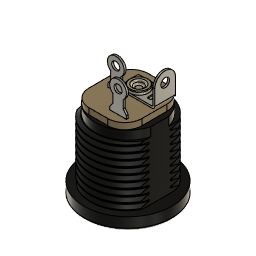
DC jack (Autodesk Fusion 360 design; units mm, degrees)
Autodesk Fusion 360 part; units mm, degrees
note: some values were not read from the file. Chosen so that the rebuilt part matches the saved one: which pieces of a blend or face edit are solid. Set by a fixed rule: which sketch regions a step uses.
sketch "Sketch1" plane through (0, 0, 0) normal (0, 0, 1) x (1, 0, 0)
  circle A0 centre (0, 0) radius 7.05
  line L0 (0, 0) -> (0, 7.05) construction
  circle A1 centre (0, 1.75) radius 3.2
  dimension "d1" = 14.1
  dimension "d2" = 6.4
  dimension "d3" = 2.1
  constraint coincident A0.centre L0.start
  constraint coincident A0 L0.end
  constraint vertical L0
  constraint coincident L0 A1.centre
  measures "d1" diameter of A0
  measures "d2" diameter of A1
  measures "d3" distance of L0.end A1
extrude "Extrude1" add sketch "Sketch1" along normal blind 2 contours A0 | A1 makes body 1
sketch "Sketch2" plane through (0, 0, 2) normal (0, 0, 1) x (-1, 0, 0)
  circle A0 centre (0, 0) radius 6
  constraint coincident A0.centre origin
extrude "Extrude2" add sketch "Sketch2" along normal blind 9.4 bodies 1
sketch "Sketch3" plane through (0, 0, 11.4) normal (0, 0, 1) x (-1, 0, 0)
  circle A0 centre (0, 0) radius 5.3
  dimension "d8" = 10.6
  constraint coincident A0.centre origin
  measures "d8" diameter of A0
extrude "Extrude3" add sketch "Sketch3" along normal blind 1.4 bodies 1
extrude "Extrude4" cut sketch "Sketch1" along normal blind 10.8 contours A1 bodies 1
thread "Thread1" "ISO Metric profile 12.0 M12x1 6g" major diameter 11.884 minor diameter 10.7405 pitch 1 angle 60 modelled right hand crest width 0.1426 on face at (-5.9925, 0.2991, 8.2667) crest through (-5.942, 0, 1.75) on bodies 1
sketch "Sketch4" plane through (0, 0, 12.8) normal (0, 0, 1) x (-1, 0, 0)
  line L0 (0, 0) -> (-5.1, 0) construction
  line L1 (0, 0) -> (0, -3.5) construction
  line L2 (-5.1, 0) -> (-5.1, -6.5)
  line L3 (-5.1, -6.5) -> (-9, -6.5)
  line L4 (-9, -6.5) -> (-9, 7.5)
  line L5 (-9, 7.5) -> (-5.1, 7.5)
  line L6 (-5.1, 7.5) -> (-5.1, 0)
  line L7 (5.1, 0) -> (5.1, -6.5)
  line L8 (5.1, -6.5) -> (9, -6.5)
  line L9 (9, -6.5) -> (9, 7.5)
  line L10 (9, 7.5) -> (5.1, 7.5)
  line L11 (5.1, 7.5) -> (5.1, 0)
  dimension "d13" = 5.1
  constraint coincident L0.start L1.start
  constraint horizontal L0
  constraint perpendicular L0 L1
  constraint perpendicular L0 L2
  constraint perpendicular L2 L3
  constraint perpendicular L3 L4
  constraint perpendicular L2 L5
  constraint perpendicular L0 L6
  constraint symmetric L0.end L1 L7.start
  constraint symmetric L1 L2.end L7.end
  constraint symmetric L1 L3.end L8.end
  constraint symmetric L1 L4.end L9.end
  constraint symmetric L1 L5.end L10.end
  measures "d13" distance of L0.start L0.end
extrude "Extrude5" cut sketch "Sketch4" against normal up to surface (10.8 mm away) bodies 1
sketch "Sketch5" plane through (0, 0, 12.8) normal (0, 0, 1) x (-1, 0, 0)
  circle A0 centre (0, -1.75) radius 3.2
  circle A1 centre (0, -1.75) radius 1
  line L0 (3.58, 0.05) -> (-3.58, 0.05)
  line L1 (0, -1.75) -> (0, 4.5) construction
  line L2 (2.17, 4.05) -> (2.17, 3.35)
  line L3 (-2.17, 4.05) -> (-2.17, 3.35)
  line L4 (3.58, 3.35) -> (2.17, 3.35)
  line L5 (-2.17, 3.35) -> (-3.58, 3.35)
  line L6 (-0.3, 4.05) -> (-0.3, 3.35)
  line L7 (0.3, 3.35) -> (0.3, 4.05)
  line L8 (-0.3, 3.35) -> (0.3, 3.35)
  line L9 (2.17, 4.05) -> (0.3, 4.05)
  line L10 (-0.3, 4.05) -> (-2.17, 4.05)
  line L11 (3.58, 3.35) -> (3.58, 3.05)
  line L12 (-3.58, 3.35) -> (-3.58, 3.05)
  line L13 (3.58, 0.05) -> (3.58, 0.35)
  line L14 (-3.58, 0.05) -> (-3.58, 0.35)
  line L15 (2.95, 0.05) -> (2.95, 3.35)
  line L16 (3.58, 0.35) -> (2.95, 0.35)
  line L17 (3.58, 3.05) -> (2.95, 3.05)
  line L18 (-3.58, 0.35) -> (-2.95, 0.35)
  line L19 (-2.95, 0.05) -> (-2.95, 3.35)
  line L20 (-3.58, 3.05) -> (-2.95, 3.05)
  dimension "d16" = 2
  dimension "d17" = 0.8
  dimension "d18" = 3.58
  dimension "d19" = 3.58
  dimension "d22" = 2.17
  dimension "d23" = 2.17
  dimension "d24" = 0.3
  dimension "d25" = 0.3
  dimension "d26" = 0.3
  dimension "d27" = 0.3
  dimension "d28" = 0.3
  dimension "d29" = 0.3
  dimension "d30" = 2.95
  constraint concentric A0 A1
  constraint horizontal L0
  constraint coincident A0.centre A1.centre
  constraint perpendicular L0 L1
  constraint parallel L0 L9
  constraint perpendicular L2 L4
  constraint coincident L3.end L4
  constraint perpendicular L3 L4
  constraint parallel L0 L4
  constraint collinear L4 L5
  constraint coincident L6.start L9
  constraint perpendicular L5 L6
  constraint perpendicular L7 L9
  constraint perpendicular L6 L8
  constraint collinear L9 L10
  constraint perpendicular L4 L11
  constraint perpendicular L5 L12
  constraint perpendicular L0 L13
  constraint perpendicular L0 L14
  constraint parallel L11 L15
  constraint perpendicular L15 L16
  constraint perpendicular L15 L17
  constraint symmetric L1 L11.end L12.end
  constraint symmetric L1 L13.end L14.end
  constraint symmetric L1 L16.end L18.end
  constraint symmetric L1 L17.end L20.end
  constraint coincident L0 L15.start
  constraint coincident L16.end L15
  constraint coincident L4 L15.end
  constraint coincident L17.end L15
  constraint coincident L0 L19.start
  constraint coincident L18.end L19
  constraint coincident L20.end L19
  measures "d16" diameter of A1
  measures "d17" distance of A1 L0
  measures "d18" distance of L0.end L1
  measures "d19" distance of L0.start L1
  measures "d22" distance of L1 L3.start
  measures "d23" distance of L1 L2.start
  measures "d24" distance of L1 L6
  measures "d25" distance of L1 L7
  measures "d26" distance of L4.start L11.end
  measures "d27" distance of L5.end L12.end
  measures "d28" distance of L0.start L13.end
  measures "d29" distance of L0.end L14.end
  measures "d30" distance of L1 L15
extrude "Extrude6" cut sketch "Sketch5" against normal blind 5.3 contours L0 L13 L15 L16 | L0 L14 L18 L19 | L4 L11 L15 L17 | L5 L12 L19 L20 bodies 1
extrude "Extrude7" cut sketch "Sketch5" against normal up to surface (10.8 mm away) contours A0 L0 | A0 L0 L2 L3 L4 L5 L6 L7 L8 L9 L10 L15 L19 picked at (0.0798, 0.5137) bodies 1
extrude "Extrude8" cut sketch "Sketch5" against normal up to surface (2 mm away) contours A1 bodies 1
fillet "Fillet1" radius 0.4 1 faces at (0.7783, -5.1149, 0) on bodies 1
sketch "Sketch6" plane through (0, -0.05, 0) normal (0, -1, 0) x (1, 0, 0)
  line L0 (-2.95, 2) -> (-2.6458, 2)
  line L1 (2.6458, 2) -> (2.95, 2)
  line L2 (-3.48, 7.5) -> (-3.044, 7.5)
  line L3 (0, 5) -> (0, 13.7) construction
  line L4 (-1.786, 9.95) -> (0, 9.95)
  line L5 (-1.8768, 9.8919) -> (-2.9532, 7.5581)
  line L6 (-3.58, 12.7) -> (-3.58, 7.6)
  arc A0 (-3.58, 7.6) -> (-3.48, 7.5) centre (-3.48, 7.6) ccw
  arc A1 (-3.044, 7.5) -> (-2.9532, 7.5581) centre (-3.044, 7.6) ccw
  arc A2 (-1.786, 9.95) -> (-1.8768, 9.8919) centre (-1.786, 9.85) ccw
  line L7 (-2.88, 12.8) -> (-2.88, 14.3)
  line L8 (-0.34, 12.8) -> (-0.34, 14.3)
  arc A3 (-3.48, 12.8) -> (-3.58, 12.7) centre (-3.48, 12.7) ccw
  line L9 (3.58, 12.7) -> (3.58, 7.6)
  arc A4 (3.58, 12.7) -> (3.48, 12.8) centre (3.48, 12.7) ccw
  arc A5 (3.48, 7.5) -> (3.58, 7.6) centre (3.48, 7.6) ccw
  line L10 (3.48, 7.5) -> (3.044, 7.5)
  arc A6 (2.9532, 7.5581) -> (3.044, 7.5) centre (3.044, 7.6) ccw
  line L11 (1.8768, 9.8919) -> (2.9532, 7.5581)
  arc A7 (1.8768, 9.8919) -> (1.786, 9.95) centre (1.786, 9.85) ccw
  line L12 (1.786, 9.95) -> (0, 9.95)
  line L13 (-5, 18.7) -> (6, 18.7) construction
  line L14 (-3.48, 12.8) -> (-2.88, 12.8)
  line L15 (-0.34, 12.8) -> (3.48, 12.8)
  line L16 (-1.61, 12.8) -> (-1.61, 18.7) construction
  circle A8 centre (-1.61, 17.35) radius 0.65
  line L17 (-2.435, 14.9814) -> (-2.435, 16.2814)
  line L18 (-2.435, 14.9814) -> (-2.88, 14.3)
  line L19 (-0.785, 14.9814) -> (-0.785, 16.2814)
  line L20 (-0.785, 14.9814) -> (-0.34, 14.3)
  arc A9 (-0.785, 16.2814) -> (-2.435, 16.2814) centre (-1.61, 17.35) ccw
  circle A10 centre (0, 11.6) radius 0.75
  point P0 (-3.58, 7.5)
  point P1 (-2.98, 7.5)
  point P2 (-1.85, 9.95)
  dimension "d39" = 0.6
  dimension "d40" = 1.85
  dimension "d42" = 0.1
  dimension "d43" = 0.1
  dimension "d44" = 0.1
  dimension "d45" = 0.7
  dimension "d46" = 2.54
  dimension "d47" = 0.1
  dimension "d50" = 1.3
  dimension "d51" = 0.7
  dimension "d54" = 1.5
  dimension "d55" = 1.5
  dimension "d56" = 0.825
  dimension "d57" = 1.3
  dimension "d58" = 1.5
  dimension "d59" = 1.2
  constraint coincident L3 L4.end
  constraint perpendicular L3 L4
  constraint perpendicular L2 L6
  constraint coincident P0 L2
  constraint coincident P0 L6
  constraint tangent L2 A0
  constraint tangent L6 A0
  constraint coincident P1 L2
  constraint coincident P1 L5
  constraint tangent L2 A1
  constraint tangent L5 A1
  constraint coincident P2 L4
  constraint coincident P2 L5
  constraint tangent L4 A2
  constraint tangent L5 A2
  constraint tangent L6 A3
  constraint symmetric L3 L4.end L12.end
  constraint symmetric L3 L2.start A5.start
  constraint symmetric L3 L6.end L9.end
  constraint symmetric L3 A0 A5
  constraint symmetric L3 L2.end L10.end
  constraint symmetric L3 L5.end A6.start
  constraint symmetric L3 A1 A6
  constraint symmetric L3 L4.start A7.end
  constraint symmetric L3 L5.start L11.start
  constraint symmetric L3 A2 A7
  constraint symmetric L3 A3.start A4.end
  constraint symmetric L3 L6.start L9.start
  constraint symmetric L3 A3 A4
  constraint horizontal L13
  constraint tangent A3 L14
  constraint perpendicular L8 L15
  constraint coincident L13 L16.end
  constraint perpendicular L13 L16
  constraint coincident L16 A8.centre
  constraint concentric A8 A9
  constraint coincident L16.end A9
  constraint vertical L17
  constraint symmetric L7.end L16 L8.end
  constraint symmetric L16 L17.start L19.start
  constraint symmetric L16 L17.end L19.end
  constraint coincident L3 A10.centre
  measures "d39" distance of P0 P1
  measures "d40" distance of L3 P2
  measures "d42" radius of A0
  measures "d43" radius of A1
  measures "d44" radius of A2
  measures "d45" distance of L6 L7
  measures "d46" distance of L7 L8
  measures "d47" radius of A3
  measures "d50" diameter of A8
  measures "d51" distance of L13 A8
  measures "d54" distance of L7.end L14
  measures "d55" distance of L8.end L15
  measures "d56" distance of L16 L17
  measures "d57" distance of L17.start L17.end
  measures "d58" diameter of A10
  measures "d59" distance of L15 A10.centre
extrude "Extrude9" add sketch "Sketch6" along normal blind 0.3 separate body contours L2 L4 L5 L6 A0 A1 A2 L7 L8 A3 L9 A4 A5 L10 A6 L11 A7 L12 L14 L15 L17 L18 L19 L20 A9 | A10 makes body 2
extrude "Extrude10" add sketch "Sketch6" along normal up to surface (0.5 mm away) contours A10 bodies 2
extrude "Extrude11" cut sketch "Sketch6" along normal blind 0.2 contours A10 bodies 2
fillet "Fillet2" radius 0.4 1 edges at (-0.6992, -0.55, 11.8712) on bodies 2
move_face "OffsetFaces1" offset 0.2 1 faces at (0.7491, -0.1833, 11.5626) on bodies 2
fillet "Fillet3" radius 0.4 1 edges at (-0.5128, -0.25, 11.4011) on bodies 2
fillet "Fillet4" radius 0.2 1 edges at (-0.5128, -0.05, 11.4011) on bodies 2
sketch "Sketch7" plane through (0, 0, 10.8) normal (0, 0, -1) x (1, 0, 0)
  circle A0 centre (0, -1.75) radius 1
  circle A1 centre (0, -1.75) radius 1.65
  dimension "d73" = 3.3
  constraint concentric A0 A1
  measures "d73" diameter of A1
extrude "Extrude12" add sketch "Sketch7" along normal blind 8 separate body contours A0 makes body 3
extrude "Extrude13" add sketch "Sketch7" along normal blind 1 bodies 3
fillet "Fillet5" radius 0.3 1 faces at (1.6418, 1.9143, 10.4667) on bodies 3
fillet "Fillet6" radius 1 1 faces at (0.4359, 2.1444, 2.8) on bodies 3
sketch "Sketch8" plane through (0, -3.35, 0) normal (0, 1, 0) x (-1, 0, 0)
  line L0 (-2.95, 2) -> (-2.17, 2)
  line L1 (2.17, 2) -> (2.95, 2)
  line L2 (-3.58, 7.5) -> (3.58, 7.5)
  line L3 (-3.58, 12.8) -> (3.58, 12.8)
  line L4 (-3.58, 12.8) -> (-3.58, 7.5)
  line L5 (3.58, 12.8) -> (3.58, 7.5)
  constraint perpendicular L2 L4
  constraint perpendicular L2 L5
extrude "Extrude14" add sketch "Sketch8" along normal blind 0.3 separate body makes body 4
sketch "Sketch9" plane through (0, 0, 0) normal (1, 0, 0) x (0, 1, 0)
  line L0 (-0.05, 7.6) -> (-0.05, 7.5)
  line L1 (-0.05, 12.7) -> (-0.05, 7.6)
  line L2 (-0.05, 12.8) -> (-0.05, 12.7)
  line L3 (-0.05, 12.8) -> (-0.05, 14.3)
  line L4 (-0.05, 14.9814) -> (-0.05, 14.3)
  line L5 (-0.05, 14.9814) -> (-0.05, 16.2814)
  line L6 (-0.05, 18.7) -> (-0.05, 16.2814)
  line L7 (-0.55, 11.1964) -> (-0.55, 12.0036)
  line L8 (-0.35, 12.7) -> (-0.35, 12.35)
  line L9 (-0.35, 10.85) -> (-0.35, 7.6)
  line L10 (-0.35, 12.8) -> (-0.35, 12.7)
  line L11 (-0.35, 14.3) -> (-0.35, 12.8)
  line L12 (-0.35, 14.9814) -> (-0.35, 14.3)
  line L13 (-0.35, 16.2814) -> (-0.35, 14.9814)
  line L14 (-0.35, 18.7) -> (-0.35, 16.2814)
  arc A0 (-0.55, 11.1964) -> (-0.35, 10.85) centre (-0.15, 11.1964) ccw
  arc A1 (-0.35, 12.35) -> (-0.55, 12.0036) centre (-0.15, 12.0036) ccw
  line L15 (-0.05, 18.7) -> (-0.35, 18.7)
  line L16 (-3.35, 12.8) -> (-3.05, 12.8)
  line L17 (-3.05, 12.8) -> (-3.05, 7.5)
  line L18 (-3.35, 7.5) -> (-3.35, 12.8)
  line L19 (2, 3) -> (-5, 3) construction
  line L20 (0.45, 2.5) -> (0.45, 9.9) construction
  line L21 (-0.55, 7.859) -> (-0.55, 11.9) construction
  line L22 (-3.35, 7.5) -> (-3.35, 3)
  line L23 (-0.55, 11.9) -> (-0.55, 7.859)
  arc A2 (-0.55, 7.859) -> (-0.4568, 7.6417) centre (-0.25, 7.859) ccw
  line L24 (-0.85, 11.9) -> (-0.85, 7.859)
  arc A3 (-0.85, 7.859) -> (-0.6636, 7.4243) centre (-0.25, 7.859) ccw
  line L25 (-0.55, 11.9) -> (-0.85, 11.9)
  line L26 (-3.05, 7.5) -> (-3.05, 3.65)
  arc A4 (-3.35, 3.65) -> (-2.2114, 3.2214) centre (-2.7, 3.65) ccw
  arc A5 (-3.05, 3.65) -> (-2.4369, 3.4192) centre (-2.7, 3.65) ccw
  line L27 (-0.4568, 7.6417) -> (0.2481, 6.9709)
  line L28 (-0.55, 11.6) -> (-0.55, 7.859)
  arc A6 (-0.55, 7.859) -> (-0.4568, 7.6417) centre (-0.25, 7.859) ccw
  line L29 (-0.6636, 7.4243) -> (0.0413, 6.7535)
  arc A7 (-0.85, 7.859) -> (-0.6636, 7.4243) centre (-0.25, 7.859) ccw
  line L30 (-0.85, 11.6) -> (-0.85, 7.859)
  line L31 (0.6338, 6.4451) -> (0.6338, 6.4787)
  line L32 (0.0631, 6.2692) -> (-2.4369, 3.4192)
  line L33 (-2.7981, 3.0074) -> (-2.8223, 2.9798)
  line L34 (0.2886, 6.0714) -> (-2.2114, 3.2214)
  arc A8 (0.0631, 6.2692) -> (0.0413, 6.7535) centre (-0.2, 6.5) ccw
  arc A9 (0.2886, 6.0714) -> (0.2481, 6.9709) centre (-0.2, 6.5) ccw
  line L35 (-2.4369, 3.4192) -> (-2.2114, 3.2214)
  point P0 (-0.55, 7.7)
  point P1 (0.45, 6.5)
  dimension "d84" = 9.8
  dimension "d85" = 3.8
  dimension "d86" = 0.9
  dimension "d87" = 4.2
  dimension "d88" = 3.5
  dimension "d91" = 0.3
  dimension "d94" = 0.65
  dimension "d95" = 0.3
  dimension "d116" = 1.3
  dimension "d117" = 0.3
  dimension "d118" = 0.3
  constraint horizontal L19
  constraint perpendicular L19 L20
  constraint perpendicular L19 L21
  constraint coincident L21 P0
  constraint coincident L20 P1
  constraint coincident L18.start L22.start
  constraint coincident L19 L22.end
  constraint perpendicular L19 L22
  constraint tangent L21 A2
  constraint parallel L23 L24
  constraint perpendicular L24 L25
  constraint tangent L19 A4
  constraint tangent L22 A4
  constraint concentric A4 A5
  constraint coincident L17.end L26.start
  constraint coincident L22 A4.start
  constraint concentric A2 A3
  constraint coincident P1 A9
  constraint concentric A8 A9
  constraint tangent L27 A9
  constraint tangent A2 L27
  constraint vertical L31
  constraint tangent L34 A9
  constraint tangent A4 L34
  constraint parallel L32 L34
  constraint coincident A4 L33.start
  constraint collinear L32 L33
  constraint perpendicular L34 L35
  measures "d84" distance of L16 L19
  measures "d85" distance of L18 L20
  measures "d86" distance of L16 L21.end
  measures "d87" distance of L21.end P0
  measures "d88" distance of L19 P1
  measures "d91" radius of A2
  measures "d94" radius of A4
  measures "d95" distance of A4 A5
  measures "d116" diameter of A9
  measures "d117" distance of A8 A9
extrude "Extrude15" add sketch "Sketch9" along normal mid plane 4.6 separate body contours L7 L23 A2 L24 A3 L25 L27 L28 A6 L29 A7 L30 L32 L34 A8 A9 L35 makes body 5
draft "Draft1" angle -5 neutral plane through (0, -2.4369, 3.4192) pull (0, -0.659438, -0.751759) 2 faces at (2.3, -0.75, 10.553) (-2.3, -0.75, 10.553) on bodies 5
extrude "Extrude16" add sketch "Sketch9" along normal mid plane 4.6 contours L16 L17 L18 L22 L26 A4 A5 L35 bodies 5
combine "Combine1" operation add target body 5 tool bodies 4
sketch "Sketch11" plane through (0, -3.05, 0) normal (0, 1, 0) x (-1, 0, 0)
  line L0 (-3.58, 12.8) -> (-3.58, 7.5)
  line L1 (3.58, 12.8) -> (-3.58, 12.8)
  line L2 (-3.08, 12.8) -> (-3.08, 14.3)
  line L3 (0.34, 12.8) -> (-3.48, 12.8)
  line L4 (-0.43, 12.8) -> (-0.43, 14.3)
  line L5 (-1.755, 12.8) -> (-1.755, 18.7) construction
  line L6 (5, 18.7) -> (-6, 18.7) construction
  circle A0 centre (-1.755, 17.35) radius 0.65
  line L7 (-0.93, 16.2814) -> (-0.93, 14.9814)
  line L8 (-0.93, 14.9814) -> (-0.43, 14.3)
  line L9 (-2.58, 16.2814) -> (-2.58, 14.9814)
  line L10 (-2.58, 14.9814) -> (-3.08, 14.3)
  arc A1 (-0.93, 16.2814) -> (-2.58, 16.2814) centre (-1.755, 17.35) ccw
  line L11 (-0.33, 12.8) -> (0, 12.8)
  dimension "d105" = 0.5
  dimension "d106" = 1.5
  dimension "d108" = 1.3
  dimension "d109" = 0.7
  dimension "d110" = 0.825
  dimension "d111" = 1.3
  constraint perpendicular L1 L2
  constraint coincident L6 L5.end
  constraint coincident L5 A0.centre
  constraint concentric A0 A1
  constraint coincident L5.end A1
  constraint parallel L5 L7
  constraint symmetric L4.end L5 L2.end
  constraint symmetric L5 L7.end L9.end
  constraint symmetric L5 L7.start L9.start
  constraint midpoint L1 L11.end
  constraint parallel L2 L4
  constraint coincident L1 L2.start
  constraint coincident L1 L4.start
  measures "d105" distance of L0 L2
  measures "d106" distance of L2.end L3
  measures "d108" diameter of A0
  measures "d109" distance of L6 A0
  measures "d110" distance of L5 L7
  measures "d111" distance of L7.end L7.start
extrude "Extrude17" add sketch "Sketch11" against normal up to surface (0.3 mm away) bodies 5
sketch "Sketch12" plane through (0, 0, 12.8) normal (0, 0, 1) x (-1, 0, 0)
  circle A0 centre (0, -1.75) radius 1
  arc A1 (-5.1, -1.4422) -> (5.1, -1.4422) centre (0, 0) ccw
  line L0 (-5.1, 1.4422) -> (-5.1, -1.4422)
  line L1 (5.1, -1.4422) -> (5.1, 1.4422)
  arc A2 (5.1, 1.4422) -> (-5.1, 1.4422) centre (0, 0) ccw
  line L2 (0, -1.75) -> (0, 7) construction
  line L3 (1.5, -4.75) -> (-1.5, -4.75)
  line L4 (4.25, -2) -> (4.25, 2)
  line L5 (0, 0) -> (-2.7166, 0) construction
  line L6 (1.5, 4.75) -> (-1.5, 4.75)
  line L7 (-4.25, -2) -> (-4.25, 2)
  arc A3 (1.5, -4.75) -> (4.25, -2) centre (1.5, -2) ccw
  arc A4 (-4.25, -2) -> (-1.5, -4.75) centre (-1.5, -2) ccw
  arc A5 (-1.5, 4.75) -> (-4.25, 2) centre (-1.5, 2) ccw
  arc A6 (4.25, 2) -> (1.5, 4.75) centre (1.5, 2) ccw
  line L8 (0, -1.75) -> (-3, -1.75) construction
  line L9 (-2, -1.75) -> (-2, -2.55)
  line L10 (-2, -2.55) -> (-2.7, -2.55)
  line L11 (-2.7, -2.55) -> (-2.7, -0.95)
  line L12 (-2, -0.95) -> (-2.7, -0.95)
  line L13 (-2, -1.75) -> (-2, -0.95)
  point P0 (0, -1.75)
  dimension "d121" = 2
  dimension "d122" = 0.85
  dimension "d123" = 2.75
  dimension "d128" = 0.8
  dimension "d130" = 1
  dimension "d131" = 0.7
  dimension "d132" = 1.6
  constraint coincident P0 A0.centre
  constraint vertical L2
  constraint vertical L4
  constraint coincident A1.centre A2.centre
  constraint perpendicular L2 L5
  constraint tangent L4 A3
  constraint tangent L3 A3
  constraint tangent L7 A4
  constraint tangent L3 A4
  constraint equal A3 A4
  constraint tangent L6 A5
  constraint tangent L7 A5
  constraint equal A3 A5
  constraint tangent L6 A6
  constraint tangent L4 A6
  constraint equal A3 A6
  constraint perpendicular L2 L8
  constraint coincident L8 L9.start
  constraint perpendicular L8 L9
  constraint perpendicular L9 L10
  constraint perpendicular L10 L11
  constraint symmetric L8 L9.start L13.start
  constraint symmetric L8 L9.end L12.start
  constraint symmetric L8 L10.end L11.end
  measures "d121" distance of A0 L3
  measures "d122" distance of L1 L4
  measures "d123" radius of A3
  measures "d128" distance of L8 L9.end
  measures "d130" distance of A0 L9
  measures "d131" distance of L9.end L10.end
  measures "d132" distance of L10.end L11.end
extrude "Extrude18" add sketch "Sketch12" along normal blind 1 separate body contours L3 L4 L6 L7 A3 A4 A5 A6 makes body 6
combine "Combine2" operation cut target body 6 tool bodies 2 5 keep tools
move_face "OffsetFaces2" offset -0.025 4 faces at (-0.34, -0.15, 13.1333) (-2.0333, -0.05, 13.1333) (-2.88, -0.15, 13.1333) (-2.0333, -0.35, 13.1333) on bodies 6
move_face "OffsetFaces3" offset -0.025 4 faces at (0.43, -3.15, 13.1333) (2.1967, -3.35, 13.4667) (2.1967, -3.05, 13.4667) (3.08, -3.15, 13.1333) on bodies 6
sketch "Sketch13" plane through (0, 0, 13.8) normal (0, 0, 1) x (-1, 0, 0)
  circle A0 centre (0, -1.75) radius 1
  line L0 (-2, -0.95) -> (-2, -2.55)
  line L1 (-2, -2.55) -> (-2.7, -2.55)
  line L2 (-2.7, -2.55) -> (-2.7, -0.95)
  line L3 (-2.7, -0.95) -> (-2, -0.95)
  circle A1 centre (0, -1.75) radius 1.085 construction
  line L4 (0.135, -0.235) -> (-4.065, -0.235)
  line L5 (1.885, -1.985) -> (1.885, -3.565)
  line L6 (1.885, -3.565) -> (-4.065, -3.565)
  line L7 (-4.065, -3.565) -> (-4.065, -0.235)
  line L8 (-2.425, -0.975) -> (-2.275, -0.975)
  line L9 (-2.025, -1.225) -> (-2.025, -2.275)
  line L10 (-2.275, -2.525) -> (-2.425, -2.525)
  line L11 (-2.675, -2.275) -> (-2.675, -1.225)
  arc A2 (-2.275, -2.525) -> (-2.025, -2.275) centre (-2.275, -2.275) ccw
  arc A3 (-2.675, -2.275) -> (-2.425, -2.525) centre (-2.425, -2.275) ccw
  arc A4 (-2.425, -0.975) -> (-2.675, -1.225) centre (-2.425, -1.225) ccw
  arc A5 (-2.025, -1.225) -> (-2.275, -0.975) centre (-2.275, -1.225) ccw
  arc A6 (1.885, -1.985) -> (0.135, -0.235) centre (0.135, -1.985) ccw
  dimension "d133" = 2.17
  dimension "d134" = 0.43
  dimension "d135" = 0.8
  dimension "d136" = 3.33
  dimension "d137" = 5.95
  dimension "d139" = 0.25
  dimension "d140" = 1.75
  constraint concentric A0 A1
  constraint horizontal L4
  constraint perpendicular L4 L5
  constraint perpendicular L5 L6
  constraint perpendicular L6 L7
  constraint parallel L3 L8
  constraint parallel L0 L9
  constraint parallel L1 L10
  constraint parallel L2 L11
  constraint tangent L9 A2
  constraint tangent L10 A2
  constraint tangent L10 A3
  constraint tangent L11 A3
  constraint equal A2 A3
  constraint tangent L8 A4
  constraint tangent L11 A4
  constraint equal A2 A4
  constraint tangent L8 A5
  constraint tangent L9 A5
  constraint equal A2 A5
  constraint tangent L5 A6
  constraint tangent L4 A6
  measures "d133" diameter of A1
  measures "d134" distance of A1 L4
  measures "d135" distance of A1 L5
  measures "d136" distance of L4 L6
  measures "d137" distance of L5 L7
  measures "d139" radius of A2
  measures "d140" radius of A6
extrude "Extrude19" add sketch "Sketch13" along normal blind 0.3 separate body contours L0 L1 L2 L3 | L4 L5 L6 L7 A6 | L8 L9 L10 L11 A2 A3 A4 A5 makes body 7
extrude "Extrude20" add sketch "Sketch13" against normal blind 0.3 contours L8 L9 L10 L11 A2 A3 A4 A5 bodies 7
fillet "Fillet7" radius 0.3 1 faces at (2.4583, 1.925, 13.5) on bodies 7
sketch "Sketch14" plane through (0, 0, 14.1) normal (0, 0, 1) x (-1, 0, 0)
  line L0 (-2.025, -1.225) -> (-2.025, -2.275)
  arc A0 (-2.025, -1.225) -> (-2.275, -0.975) centre (-2.275, -1.225) ccw
  line L1 (-2.425, -0.975) -> (-2.275, -0.975)
  arc A1 (-2.425, -0.975) -> (-2.675, -1.225) centre (-2.425, -1.225) ccw
  line L2 (-2.675, -2.275) -> (-2.675, -1.225)
  arc A2 (-2.675, -2.275) -> (-2.425, -2.525) centre (-2.425, -2.275) ccw
  line L3 (-2.275, -2.525) -> (-2.425, -2.525)
  arc A3 (-2.275, -2.525) -> (-2.025, -2.275) centre (-2.275, -2.275) ccw
  line L4 (-2.125, -1.225) -> (-2.125, -2.275)
  arc A4 (-2.275, -2.425) -> (-2.125, -2.275) centre (-2.275, -2.275) ccw
  line L5 (-2.275, -2.425) -> (-2.425, -2.425)
  arc A5 (-2.575, -2.275) -> (-2.425, -2.425) centre (-2.425, -2.275) ccw
  line L6 (-2.575, -2.275) -> (-2.575, -1.225)
  arc A6 (-2.425, -1.075) -> (-2.575, -1.225) centre (-2.425, -1.225) ccw
  line L7 (-2.425, -1.075) -> (-2.275, -1.075)
  arc A7 (-2.125, -1.225) -> (-2.275, -1.075) centre (-2.275, -1.225) ccw
  dimension "d147" = 0.1
extrude "Extrude21" cut sketch "Sketch14" against normal blind 0.3 contours L4 A4 L5 A5 L6 A6 L7 A7 bodies 7
fillet "Fillet8" radius 0.2 1 faces at (2.425, 1.925, 13.8) on bodies 7
fillet "Fillet9" radius 0.1 8 edges at (2.35, 2.425, 14.1) (2.5311, 2.3811, 14.1) (2.575, 1.75, 14.1) (2.5311, 1.1189, 14.1) (2.35, 1.075, 14.1) (2.1689, 1.1189, 14.1) (2.125, 1.75, 14.1) (2.1689, 2.3811, 14.1) on bodies 7
sketch "Sketch16" plane through (4.065, 0, 0) normal (1, 0, 0) x (0, 1, 0)
  line L0 (0.235, 13.8) -> (3.565, 13.8)
  line L1 (3.565, 13.8) -> (3.565, 14.1)
  line L2 (3.565, 14.1) -> (0.235, 14.1)
  line L3 (0.235, 14.1) -> (0.235, 13.8)
  line L4 (0.235, 13.8) -> (0.235, 16.735)
  line L5 (3.565, 16.735) -> (3.565, 13.8)
  arc A0 (3.565, 16.735) -> (0.235, 16.735) centre (1.9, 16.735) ccw
  circle A1 centre (1.9, 16.735) radius 0.7
  dimension "d155" = 1.665
  dimension "d156" = 1.4
  constraint coincident L0.start L3.end
  constraint perpendicular L0 L4
  constraint coincident L0.end L1.start
  constraint perpendicular L2 L5
  constraint tangent L4 A0
  constraint concentric A0 A1
  measures "d155" radius of A0
  measures "d156" diameter of A1
extrude "Extrude22" add sketch "Sketch16" against normal blind 0.3 contours L2 L4 L5 A0 bodies 7
fillet "Fillet10" radius 0.45 1 edges at (4.065, 1.9, 13.8) on bodies 7
fillet "Fillet10" radius 0.15 1 edges at (3.765, 1.9, 14.1) on bodies 7
fillet "Fillet11" radius 0.1 1 edges at (-1.885, 3.565, 13.95) on bodies 7
extrude "Extrude23" add sketch "Sketch7" against normal up to surface (3.3 mm away) contours A0 bodies 3
sketch "Sketch17" plane through (0, 0, 14.1) normal (0, 0, 1) x (-1, 0, 0)
  line L0 (0.135, -0.235) -> (-3.615, -0.235)
  circle A0 centre (0, -1.75) radius 1
  circle A1 centre (0, -1.75) radius 1.515
  constraint concentric A0 A1
  constraint tangent L0 A1
extrude "Extrude24" add sketch "Sketch17" along normal blind 0.5 contours A0 | A1 bodies 3
sketch "Sketch18" plane through (0, 0, 14.6) normal (0, 0, 1) x (-1, 0, 0)
  circle A0 centre (0, -1.75) radius 1.515
  circle A1 centre (0, -1.75) radius 0.75
  dimension "d169" = 1.5
  constraint concentric A0 A1
  measures "d169" diameter of A1
extrude "Extrude25" cut sketch "Sketch18" against normal blind 0.5 contours A1 bodies 3
fillet "Fillet12" radius 0.3 1 faces at (-0.5135, 1.8864, 14.1) on bodies 3
fillet "Fillet13" radius 0.3 1 edges at (0.6992, 1.4788, 14.6) on bodies 3
fillet "Fillet14" radius 0.1 1 edges at (1.4125, 2.2978, 14.6) on bodies 3
equation "d6 = 10.8 mm - 1.4 mm"
equation "d13 = ( 10.2 / 2 ) * 1 mm"
equation "d18 = ( 7.16 / 2 ) * 1 mm"
equation "d19 = d18"
equation "d22 = ( 4.34 / 2 ) * 1 mm"
equation "d23 = d22"
equation "d25 = d24"
equation "d30 = ( 5.9 / 2 ) * 1 mm"
equation "d40 = ( 3.7 / 2 ) * 1 mm"
equation "d56 = ( 1.65 / 2 ) * 1 mm"
equation "d101 = ( 4.6 / 2 ) * 1 mm"
equation "d110 = ( 1.65 / 2 ) * 1 mm"
equation "d128 = ( 1.6 / 2 ) * 1 mm"
equation "d155 = ( 3.33 / 2 ) * 1 mm"
